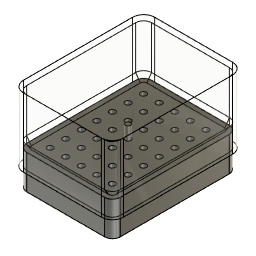
Blade Holder v3 (Autodesk Fusion 360 design; units mm, degrees)
Autodesk Fusion 360 part; units mm, degrees
sketch "Sketch1" plane through (0, 0, 0) normal (0, 0, 1) x (1, 0, 0) in component "Blades"
  circle A0 centre (0, 0) radius 1.595
  dimension "d1" = 3.19
  constraint coincident A0.centre origin
  measures "d1" diameter of A0
extrude "Extrude1" add sketch "Sketch1" along normal blind 28.3 makes body 1 in component "Blades"
sketch "Sketch1 (2)" plane through (0, 0, 0) normal (0, 0, 1) x (1, 0, 0) in component "Holder"
  circle A0 centre (0, 0) radius 1.845
  circle A1 centre (-20, -30) radius 1.845
  circle A2 centre (-10, -30) radius 1.845
  circle A3 centre (-20, -20) radius 1.845
  circle A4 centre (-10, -20) radius 1.845
  circle A5 centre (-20, -10) radius 1.845
  line L0 (-30, -40) -> (30, -40)
  line L1 (30, -40) -> (30, 40)
  line L2 (30, 40) -> (-30, 40)
  line L3 (-30, 40) -> (-30, -40)
  circle A6 centre (0, -30) radius 1.845
  circle A7 centre (10, -30) radius 1.845
  circle A8 centre (20, -30) radius 1.845
  circle A9 centre (0, -20) radius 1.845
  circle A10 centre (10, -20) radius 1.845
  circle A11 centre (20, -20) radius 1.845
  circle A12 centre (-10, -10) radius 1.845
  circle A13 centre (0, -10) radius 1.845
  circle A14 centre (10, -10) radius 1.845
  circle A15 centre (20, -10) radius 1.845
  circle A16 centre (-20, 0) radius 1.845
  circle A17 centre (-10, 0) radius 1.845
  circle A18 centre (10, 0) radius 1.845
  circle A19 centre (20, 0) radius 1.845
  circle A20 centre (-20, 10) radius 1.845
  circle A21 centre (-10, 10) radius 1.845
  circle A22 centre (0, 10) radius 1.845
  circle A23 centre (10, 10) radius 1.845
  circle A24 centre (20, 10) radius 1.845
  circle A25 centre (-20, 20) radius 1.845
  circle A26 centre (-10, 20) radius 1.845
  circle A27 centre (0, 20) radius 1.845
  circle A28 centre (10, 20) radius 1.845
  circle A29 centre (20, 20) radius 1.845
  circle A30 centre (-20, 30) radius 1.845
  circle A31 centre (-10, 30) radius 1.845
  circle A32 centre (0, 30) radius 1.845
  circle A33 centre (10, 30) radius 1.845
  circle A34 centre (20, 30) radius 1.845
  line L4 (30, 0) -> (0, 0) construction
  line L5 (0, 0) -> (0, 40) construction
  dimension "d8" = 10
  dimension "d9" = 10
  dimension "d12" = 3.69
  dimension "d24" = 60
  dimension "d25" = 80
  constraint horizontal L0
  constraint vertical L1
  constraint horizontal L2
  constraint vertical L3
  constraint coincident A0.centre L4.end
  constraint midpoint L1 L4.start
  constraint midpoint L2 L5.end
  constraint perpendicular L2 L5
  constraint perpendicular L1 L4
  measures "d12" diameter of A0
  measures "d24" distance of L1 L3
  measures "d25" distance of L0.end L1.end
extrude "Extrude1'" add sketch "Sketch1 (2)" along normal blind 20 separate body makes body 2 in component "Holder"
sketch "Sketch2" plane through (0, 0, 0) normal (0, 0, -1) x (1, 0, 0) in component "Holder"
  circle A0 centre (-10, -10) radius 1.845 construction
  circle A1 centre (-20, -10) radius 1.845 construction
  circle A2 centre (20, 0) radius 1.845 construction
  circle A3 centre (10, 0) radius 1.845 construction
  circle A4 centre (-10, 0) radius 1.845 construction
  circle A5 centre (10, 20) radius 1.845 construction
  circle A6 centre (20, 20) radius 1.845 construction
  circle A7 centre (-10, 10) radius 1.845 construction
  circle A8 centre (0, 10) radius 1.845 construction
  circle A9 centre (10, 10) radius 1.845 construction
  circle A10 centre (-20, 0) radius 1.845 construction
  circle A11 centre (20, 10) radius 1.845 construction
  circle A12 centre (0, 20) radius 1.845 construction
  circle A13 centre (0, -10) radius 1.845 construction
  circle A14 centre (10, -10) radius 1.845 construction
  circle A15 centre (20, -10) radius 1.845 construction
  circle A16 centre (-20, -20) radius 1.845 construction
  circle A17 centre (-10, -20) radius 1.845 construction
  circle A18 centre (0, -20) radius 1.845 construction
  circle A19 centre (10, -20) radius 1.845 construction
  circle A20 centre (20, -20) radius 1.845 construction
  circle A21 centre (-20, -30) radius 1.845 construction
  circle A22 centre (-10, -30) radius 1.845 construction
  circle A23 centre (0, -30) radius 1.845 construction
  circle A24 centre (10, -30) radius 1.845 construction
  circle A25 centre (20, -30) radius 1.845 construction
  circle A26 centre (10, 30) radius 1.845 construction
  circle A27 centre (-20, 30) radius 1.845 construction
  circle A28 centre (20, 30) radius 1.845 construction
  circle A29 centre (0, 30) radius 1.845 construction
  circle A30 centre (0, 0) radius 1.845 construction
  circle A31 centre (-10, 30) radius 1.845 construction
  circle A32 centre (-10, 20) radius 1.845 construction
  circle A33 centre (-20, 20) radius 1.845 construction
  circle A34 centre (-20, 10) radius 1.845 construction
  line L0 (-30, 40) -> (-30, -40)
  line L1 (-30, -40) -> (30, -40)
  line L2 (30, -40) -> (30, 40)
  line L3 (30, 40) -> (-30, 40)
extrude "Extrude2" add sketch "Sketch2" along normal blind 2 bodies 2 in component "Holder"
fillet "Fillet2" radius 5 4 edges at (-30, -40, 9) (30, -40, 9) (-30, 40, 9) (30, 40, 9) on bodies 2 in component "Holder"
ref_plane "WorkPlane1" through (0, 0, 10) normal (0, 0, 1) x (1, 0, 0) in component "Holder"
sketch "Sketch3" plane through (0, 0, 10) normal (0, 0, 1) x (1, 0, 0) in component "Holder"
  arc A0 (30, 35) -> (25, 40) centre (25, 35) ccw construction
  line L0 (25, 40) -> (-25, 40) construction
  arc A1 (-25, 40) -> (-30, 35) centre (-25, 35) ccw construction
  line L1 (-30, 35) -> (-30, -35) construction
  arc A2 (-30, -35) -> (-25, -40) centre (-25, -35) ccw construction
  line L2 (-25, -40) -> (25, -40) construction
  arc A3 (25, -40) -> (30, -35) centre (25, -35) ccw construction
  line L3 (30, -35) -> (30, 35) construction
  circle A4 centre (20, 0) radius 1.845 construction
  circle A5 centre (-20, 10) radius 1.845 construction
  circle A6 centre (-10, 10) radius 1.845 construction
  circle A7 centre (0, 0) radius 1.845 construction
  circle A8 centre (-20, -30) radius 1.845 construction
  circle A9 centre (-10, -30) radius 1.845 construction
  circle A10 centre (-20, -20) radius 1.845 construction
  circle A11 centre (-10, -20) radius 1.845 construction
  circle A12 centre (10, 0) radius 1.845 construction
  circle A13 centre (-10, 0) radius 1.845 construction
  circle A14 centre (-20, 0) radius 1.845 construction
  circle A15 centre (10, -10) radius 1.845 construction
  circle A16 centre (20, -10) radius 1.845 construction
  circle A17 centre (0, -10) radius 1.845 construction
  circle A18 centre (-10, -10) radius 1.845 construction
  circle A19 centre (0, 20) radius 1.845 construction
  circle A20 centre (10, 20) radius 1.845 construction
  circle A21 centre (20, 20) radius 1.845 construction
  circle A22 centre (-20, 30) radius 1.845 construction
  circle A23 centre (-10, 30) radius 1.845 construction
  circle A24 centre (0, 30) radius 1.845 construction
  circle A25 centre (-20, 20) radius 1.845 construction
  circle A26 centre (10, 30) radius 1.845 construction
  circle A27 centre (20, 30) radius 1.845 construction
  circle A28 centre (20, 10) radius 1.845 construction
  circle A29 centre (0, 10) radius 1.845 construction
  circle A30 centre (10, 10) radius 1.845 construction
  circle A31 centre (-10, 20) radius 1.845 construction
  circle A32 centre (10, -30) radius 1.845 construction
  circle A33 centre (10, -20) radius 1.845 construction
  circle A34 centre (-20, -10) radius 1.845 construction
  circle A35 centre (20, -20) radius 1.845 construction
  circle A36 centre (0, -30) radius 1.845 construction
  circle A37 centre (0, -20) radius 1.845 construction
  circle A38 centre (20, -30) radius 1.845 construction
  line L4 (-25, -40.1) -> (25, -40.1)
  arc A39 (25, -40.1) -> (30.1, -35) centre (25, -35) ccw
  line L5 (30.1, -35) -> (30.1, 35)
  arc A40 (30.1, 35) -> (25, 40.1) centre (25, 35) ccw
  line L6 (25, 40.1) -> (-25, 40.1)
  arc A41 (-25, 40.1) -> (-30.1, 35) centre (-25, 35) ccw
  line L7 (-30.1, 35) -> (-30.1, -35)
  arc A42 (-30.1, -35) -> (-25, -40.1) centre (-25, -35) ccw
  arc A43 (25, -42.1) -> (32.1, -35) centre (25, -35) ccw
  line L8 (32.1, -35) -> (32.1, 35)
  arc A44 (32.1, 35) -> (25, 42.1) centre (25, 35) ccw
  line L9 (25, 42.1) -> (-25, 42.1)
  arc A45 (-25, 42.1) -> (-32.1, 35) centre (-25, 35) ccw
  line L10 (-32.1, 35) -> (-32.1, -35)
  arc A46 (-32.1, -35) -> (-25, -42.1) centre (-25, -35) ccw
  line L11 (-25, -42.1) -> (25, -42.1)
  dimension "d35" = 0.1
  dimension "d36" = 2.1
extrude "Extrude3" add sketch "Sketch3" along normal up to surface (42 mm away) separate body makes body 3 in component "Holder"
sketch "Sketch5" plane through (0, 0, 52) normal (0, 0, 1) x (-1, 0, 0) in component "Holder"
  arc A0 (30.1, 35) -> (25, 40.1) centre (25, 35) ccw construction
  line L0 (30.1, 35) -> (30.1, -35) construction
  arc A1 (25, -40.1) -> (30.1, -35) centre (25, -35) ccw construction
  line L1 (25, -40.1) -> (-25, -40.1) construction
  arc A2 (-30.1, -35) -> (-25, -40.1) centre (-25, -35) ccw construction
  line L2 (-30.1, -35) -> (-30.1, 35) construction
  arc A3 (-25, 40.1) -> (-30.1, 35) centre (-25, 35) ccw construction
  line L3 (-25, 40.1) -> (25, 40.1) construction
  line L4 (25, 42.1) -> (-25, 42.1)
  arc A4 (-25, 42.1) -> (-32.1, 35) centre (-25, 35) ccw
  line L5 (-32.1, 35) -> (-32.1, -35)
  arc A5 (-32.1, -35) -> (-25, -42.1) centre (-25, -35) ccw
  line L6 (-25, -42.1) -> (25, -42.1)
  arc A6 (25, -42.1) -> (32.1, -35) centre (25, -35) ccw
  line L7 (32.1, -35) -> (32.1, 35)
  arc A7 (32.1, 35) -> (25, 42.1) centre (25, 35) ccw
extrude "Extrude4" add sketch "Sketch5" along normal blind 2 bodies 3 in component "Holder"
ref_plane "WorkPlane2" through (0, 0, 32) normal (-1, 0, 0) x (0, -1, 0) in component "Holder"
sketch "Sketch7" plane through (0, 0, 26) normal (-1, 0, 0) x (0, 1, 0) in component "Holder"
  line L0 (40, 6) -> (35, 6) construction
  line L1 (40, 6) -> (35, 6) construction
  line L2 (35, 6) -> (-35, 6) construction
  line L3 (-35, 6) -> (-40, 6) construction
  line L4 (-35, 6) -> (-40, 6) construction
  line L5 (-35, 6) -> (35, 6) construction
  line L6 (1.845, 6) -> (-1.845, 6) construction
  line L7 (11.845, 6) -> (8.155, 6) construction
  line L8 (11.845, 6) -> (8.155, 6) construction
  line L9 (1.845, 6) -> (-1.845, 6) construction
  line L10 (-28.155, 6) -> (-31.845, 6) construction
  line L11 (-28.155, 6) -> (-31.845, 6) construction
  line L12 (-18.155, 6) -> (-21.845, 6) construction
  line L13 (-18.155, 6) -> (-21.845, 6) construction
  line L14 (1.845, 6) -> (-1.845, 6) construction
  line L15 (1.845, 6) -> (-1.845, 6) construction
  line L16 (1.845, 6) -> (-1.845, 6) construction
  line L17 (-8.155, 6) -> (-11.845, 6) construction
  line L18 (-8.155, 6) -> (-11.845, 6) construction
  line L19 (-8.155, 6) -> (-11.845, 6) construction
  line L20 (-8.155, 6) -> (-11.845, 6) construction
  line L21 (21.845, 6) -> (18.155, 6) construction
  line L22 (21.845, 6) -> (18.155, 6) construction
  line L23 (21.845, 6) -> (18.155, 6) construction
  line L24 (31.845, 6) -> (28.155, 6) construction
  line L25 (31.845, 6) -> (28.155, 6) construction
  line L26 (31.845, 6) -> (28.155, 6) construction
  line L27 (21.845, 6) -> (18.155, 6) construction
  line L28 (31.845, 6) -> (28.155, 6) construction
  line L29 (31.845, 6) -> (28.155, 6) construction
  line L30 (11.845, 6) -> (8.155, 6) construction
  line L31 (11.845, 6) -> (8.155, 6) construction
  line L32 (11.845, 6) -> (8.155, 6) construction
  line L33 (21.845, 6) -> (18.155, 6) construction
  line L34 (-28.155, 6) -> (-31.845, 6) construction
  line L35 (-18.155, 6) -> (-21.845, 6) construction
  line L36 (-8.155, 6) -> (-11.845, 6) construction
  line L37 (-18.155, 6) -> (-21.845, 6) construction
  line L38 (-28.155, 6) -> (-31.845, 6) construction
  line L39 (-18.155, 6) -> (-21.845, 6) construction
  line L40 (-28.155, 6) -> (-31.845, 6) construction
  line L41 (-37.1, 6) -> (-40.1, 1.7156)
  line L42 (-40.1, 1.7156) -> (-40.1, 6)
  line L43 (-40.1, 6) -> (-37.1, 6)
  dimension "d43" = 35
  dimension "d44" = 0.1
  dimension "d45" = 3
  constraint horizontal L43
  constraint vertical L42
  constraint coincident L4 L41.start
  measures "d43" angle of L41 L42
  measures "d44" distance of L3.end L42
  measures "d45" distance of L42.end L41.start
sweep "Sweep1" add profiles "Sketch7" along 8 edges at (28.5355, -38.5355, 20) (30, 0, 20) (28.5355, 38.5355, 20) (0, 40, 20) (-28.5355, 38.5355, 20) (-30, 0, 20) (-28.5355, -38.5355, 20) (0, -40, 20) section 1 on bodies 2 bodies 3 in component "Holder"
component "Blades" placed x (1, 0, 0) y (0, 1, 0) z (0, 0, 1) at (0, 0, 0)
component "Holder" placed x (1, 0, 0) y (0, 1, 0) z (0, 0, 1) at (0, 0, 0)
equation "d1 = blade_shaft_diameter"
equation "rows = 5"
equation "columns = 7"
equation "d6 = rows"
equation "d7 = columns"
equation "d8 = spacing"
equation "d9 = spacing"
equation "blade_shaft_diameter = 3.19 mm"
equation "blade_shaft_clearance = 0.5 mm"
equation "d12 = blade_shaft_diameter + blade_shaft_clearance"
equation "spacing = 10 mm"
equation "d24 = spacing * ( rows + 1 )"
equation "d25 = spacing * ( columns + 1 )"
equation "lid_clearance = 0.1 mm"
equation "lid_overlap = 10 mm"
equation "d34 = -lid_overlap"
equation "d35 = lid_clearance"
equation "d36 = lid_clearance + lid_thickness"
equation "lid_thickness = 2 mm"
equation "d41 = lid_thickness"
equation "d43 = 35 °"
equation "d44 = lid_clearance"
